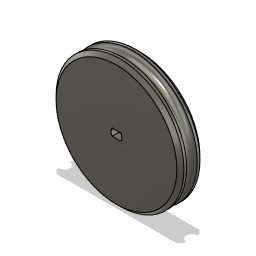
Hjul_O_ring v5 (Autodesk Fusion 360 design; units mm, degrees)
Autodesk Fusion 360 part; units mm, degrees
sketch "Sketch1" plane through (0, 0, 0) normal (0, 0, 1) x (1, 0, 0)
  circle A0 centre (0, 0) radius 1.55
  line L0 (-1.1843, 1) -> (1.1843, 1)
  line L1 (-1.1843, -1) -> (1.1843, -1)
  line L2 (0, 1) -> (0, -1) construction
  circle A1 centre (0, 0) radius 18
  dimension "d1" = 3.1
  dimension "d2" = 2
  dimension "d3" = 36
  constraint coincident A0.centre A1.centre
  constraint coincident A0 L0.start
  constraint coincident A0 L0.end
  constraint horizontal L0
  constraint coincident A0 L1.start
  constraint coincident A0 L1.end
  constraint parallel L0 L1
  constraint coincident L0 L2.start
  constraint coincident L1 L2.end
  constraint perpendicular L1 L2
  constraint midpoint A0.centre L2
  measures "d1" diameter of A0
  measures "d2" distance of L2.start L2.end
  measures "d3" diameter of A1
ref_plane "WorkPlane1" through (18, 0, 0) normal (0, 1, 0) x (-1, 0, 0)
sketch "Sketch2" plane through (18, 0, 0) normal (0, 1, 0) x (-1, 0, 0)
  circle A0 centre (0, 0) radius 1.5
  dimension "d5" = 3
  constraint coincident A0.centre origin
  measures "d5" diameter of A0
extrude "Extrude1" add sketch "Sketch1" along normal mid plane 6.5 contours A0 L0 | A0 L1 | A1
sweep "Sweep1" cut profiles "Sketch2" path "Sketch1" along A1 section 1
sketch "Sketch3" plane through (0, 0, -3.25) normal (0, 0, -1) x (-1, 0, 0)
  arc A0 (1.1843, -1) -> (1.1843, 1) centre (0, 0) ccw
  line L0 (1.1843, -1) -> (-1.1843, -1)
  arc A1 (-1.1843, 1) -> (-1.1843, -1) centre (0, 0) ccw
  line L1 (-1.1843, 1) -> (1.1843, 1)
  circle A2 centre (0, 0) radius 18
  circle A3 centre (0, 0) radius 12
  dimension "d14" = 24
  constraint concentric A0 A3
  measures "d14" diameter of A3
extrude "Extrude2" cut sketch "Sketch3" against normal blind 4.3 contours A3
chamfer "Chamfer1" distance 4.3 angle 45 1 edges at (11.1879, 4.3394, -3.25)
sketch "Sketch4" plane through (0, 0, 1.05) normal (0, 0, -1) x (-1, 0, 0)
  arc A0 (1.1843, -1) -> (1.1843, 1) centre (0, 0) ccw
  line L0 (1.1843, -1) -> (-1.1843, -1)
  arc A1 (-1.1843, 1) -> (-1.1843, -1) centre (0, 0) ccw
  line L1 (-1.1843, 1) -> (1.1843, 1)
  circle A2 centre (0, 0) radius 2.3
  circle A3 centre (0, 0) radius 12
  dimension "d23" = 4.6
  constraint concentric A0 A2
  measures "d23" diameter of A2
extrude "Extrude4" add sketch "Sketch4" along normal blind 0.8 contours A2
chamfer "Chamfer3" distance 1 angle 45 2 edges at (-16.7819, -6.5091, 3.25) (-16.7819, 6.5091, -3.25)
equation "d6 = ( ( 5.9 / 2 ) * 1 mm ) + 0.3 mm"
equation "d15 = -3.5 mm - 0.8 mm"
named bodies: "Hjul"
